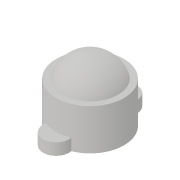
# Autodesk Inventor part: caster ball 1 2 inch
Saved by Autodesk Inventor 2018 (Build 220112000, 112)
## iProperties
Created: 2019-02-07
Part Number: caster ball 1 2 inch
Material: Generic
Document SubType Name: Modeling
Designer: ball
Density: 1 g/cm^3
Appearance: Default
Author: ball
Autodesk Inventor part; units mm, degrees
ref_plane "YZ Plane" through (0, 0, 0) normal (1, 0, 0) x (0, 1, 0)
ref_plane "XZ Plane" through (0, 0, 0) normal (0, 1, 0) x (-1, 0, 0)
sketch "Sketch1" plane through (0, 0, 0) normal (0, 1, 0) x (-1, 0, 0)
  circle A0 centre (0, 0) radius 7.366
  dimension "d0" = 14.732
  constraints: 1 centre point, 1 coincident
  measures "d0" diameter of A0
extrude "Extrusion1" add sketch "Sketch1" along normal blind 8.89
ref_plane "Work Plane1" through (0, 7.112, 0) normal (0, -1, 0) x (1, 0, 0)
sketch "Sketch2" plane through (0, 7.112, 0) normal (0, -1, 0) x (1, 0, 0)
  arc A0 (-6.35, 0) -> (6.35, 0) centre (0, 0) ccw
  circle A1 centre (0, 0) radius 7.366 construction
  line L0 (-7.366, 0) -> (7.366, 0) construction
  line L1 (-6.35, 0) -> (6.35, 0)
  dimension "d4" = 12.7
  constraints: 4 end point, 4 point on circle, 2 point on line, 1 centre point, 1 coincident, 1 horizontal
  measures "d4" diameter of A0
revolve "Revolution1" add sketch "Sketch2" angle 360 about axis through (-7.366, 7.112, 0) along (1, 0, 0)
sketch "Sketch3" plane through (0, 0, 0) normal (0, -1, 0) x (1, 0, 0)
  line L0 (0, 7.3938) -> (0, -7.366) construction
  circle A0 centre (0, 0) radius 7.366 construction
  circle A1 centre (0, 7.3938) radius 2.794
  circle A2 centre (0, -7.366) radius 2.794
  dimension "d6" = 5.588
  dimension "d7" = 5.588
  constraints: 2 centre point, 2 coincident, 2 end point, 1 vertical, 1 vertical alignment, 1 other
  measures "d6" diameter of A1
  measures "d7" diameter of A2
extrude "Extrusion2" add sketch "Sketch3" against normal blind 2.54
body "Solid1"
